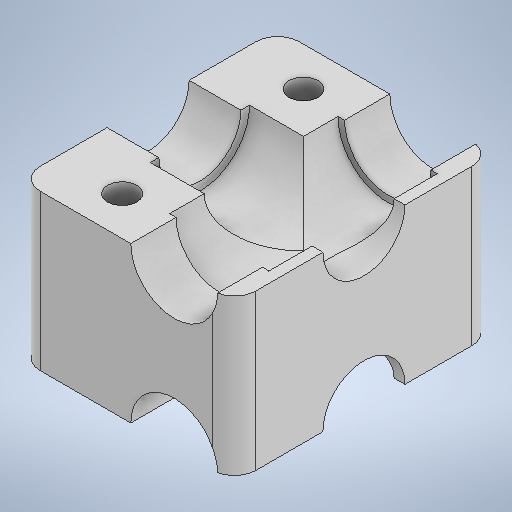
# Autodesk Inventor part: Valve Block Middle
Saved by Autodesk Inventor 2025 (Build 290162000, 162)
## iProperties
Created: 2025-04-03
Part Number: Valve Block Middle
Material: Generic
Document SubType Name: Modeling
Designer: Caleb Fangmeier
Density: 1 g/cm^3
Appearance: Default
Author: Caleb Fangmeier
Autodesk Inventor part; units mm, degrees
ref_plane "XZ Plane" through (0, 0, 0) normal (0, 1, 0) x (-1, 0, 0)
ref_plane "XY Plane" through (0, 0, 0) normal (0, 0, 1) x (1, 0, 0)
sketch "Sketch1" plane through (0, 0, 0) normal (0, 1, 0) x (-1, 0, 0)
  line L0 (-25, 30) -> (25, 30)
  line L1 (25, 30) -> (25, -30)
  line L2 (25, -30) -> (-25, -30)
  line L3 (-25, -30) -> (-25, 30)
  line L4 (-25, 30) -> (25, -30) construction
  line L5 (25, 30) -> (-25, -30) construction
  point P0 (0, 0)
  dimension "d0" = 50
  dimension "d1" = 60
  constraints: 12 end point, 2 midpoint, 2 parallel, 1 horizontal, 1 perpendicular
  measures "d0" distance of L1.end L2.end
  measures "d1" distance of L0.end L1.end
extrude "Extrusion1" add sketch "Sketch1" along normal blind 18
sketch "Sketch2" plane through (25, 0, 30) normal (1, 0, 0) x (0, 0, -1)
  line L0 (60, 18) -> (0, 18) projected
  circle A0 centre (30, 18) radius 9.5
  point P0 (30, 0)
  point P1 (20.5, 18)
  point P2 (39.5, 18)
  dimension "d4" = 19
  constraints: 1 centre point, 1 midpoint
  measures "d4" diameter of A0
extrude "Extrusion2" cut sketch "Sketch2" against normal through all contours A0 L0 picked at (28.8771, 15.0391)
sketch "Sketch3" plane through (25, 0, -30) normal (0, 0, -1) x (-1, 0, 0)
  line L0 (0, 18) -> (50, 18) projected
  circle A0 centre (14, 18) radius 10
  point P0 (25, 0)
  point P1 (24, 18)
  point P2 (4, 18)
  dimension "d7" = 20
  dimension "d8" = 14
  constraints: 1 centre point, 1 point on line
  measures "d7" diameter of A0
  measures "d8" distance of L0.start A0.centre
extrude "Extrusion3" cut sketch "Sketch3" against normal through all contours L0 A0 picked at (12.1065, 15.2567)
sketch "Sketch4" plane through (0, 0, 0) normal (0, 0, 1) x (1, 0, 0)
  arc A0 (1, 18) -> (21, 18) centre (11, 18) ccw projected
  circle A1 centre (11, 18) radius 11.5
  point P0 (0, 0)
  dimension "d11" = 23
  constraints: 1 centre point, 1 coincident
  measures "d11" diameter of A1
extrude "Extrusion4" cut sketch "Sketch4" along normal mid plane 39
ref_plane "Work Plane2" through (11, 18, -30) normal (1, 0, 0) x (0, 1, 0)
sketch "Sketch5" plane through (11, 18, -30) normal (1, 0, 0) x (0, 1, 0)
  arc A0 (0, 39.5) -> (0, 20.5) centre (0, 30) ccw projected
  circle A1 centre (0, 30) radius 11.5
  point P0 (-18, 30)
  dimension "d14" = 23
  constraints: 1 centre point, 1 coincident
  measures "d14" diameter of A1
extrude "Extrusion5" cut sketch "Sketch5" against normal blind 24
sketch "Sketch7" plane through (0, 0, 0) normal (0, -1, 0) x (1, 0, 0)
  line L0 (25, -30) -> (-25, -30) projected
  line L1 (-25, 30) -> (25, 30) projected
  line L2 (-25, -30) -> (-25, 30) projected
  point P0 (0, 0)
  point P1 (-10, -21)
  point P2 (-10, 21)
  dimension "d28" = 9
  dimension "d29" = 9
  dimension "d30" = 15
  constraints: 1 vertical alignment
  measures "d28" distance from line of L0 point (-10, -21)
  measures "d29" distance from line of point (-10, 21) L1
  measures "d30" distance from line of L2 point (-10, -21)
hole "Hole2" at (-10, 0, -21) at (-10, 0, 21) direction (0, 1, 0) diameter 6.756 end through all clearance for "Socket Head Cap Screw" size "1/4" standard "Ansi Unified Screw Threads"
fillet "Fillet1" radius 5 4 edges at (-25, 9, -30) (-25, 9, 30) (25, 9, 30) (25, 9, -30)
mirror "Mirror1" about plane through (0, 0, 0) normal (0, -1, 0)
equation "\"d28\" = d29"
body "Solid1"
